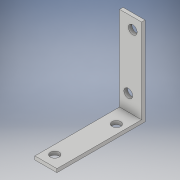
# Autodesk Inventor part: Plywood Pickle Mount Corner Bracket
Saved by Autodesk Inventor 2018 (Build 220112000, 112)
## iProperties
Created: 2018-02-14
Part Number: Plywood Pickle Mount Corner Bracket
Material: Generic
Document SubType Name: Modeling
Designer: owner
Density: 1 g/cm^3
Appearance: Default
Author: owner
Autodesk Inventor part; units mm, degrees
ref_plane "YZ Plane" through (0, 0, 0) normal (1, 0, 0) x (0, 1, 0)
ref_plane "XZ Plane" through (0, 0, 0) normal (0, 1, 0) x (-1, 0, 0)
ref_plane "XY Plane" through (0, 0, 0) normal (0, 0, 1) x (1, 0, 0)
sketch "Sketch1" plane through (0, 0, 0) normal (1, 0, 0) x (0, 1, 0)
  line L0 (0, 0) -> (0, -63.5)
  line L1 (0, -63.5) -> (63.5, -63.5)
  line L2 (63.5, -63.5) -> (63.5, -60.96)
  line L3 (0, 0) -> (2.54, 0)
  line L4 (2.54, 0) -> (2.54, -60.96)
  line L5 (2.54, -60.96) -> (63.5, -60.96)
  dimension "d0" = 63.5
  dimension "d1" = 63.5
  dimension "d2" = 2.54
  dimension "d3" = 2.54
  constraints: 12 end point, 3 perpendicular, 1 horizontal, 1 parallel, 1 vertical
  measures "d0" distance of L0.start L0.end
  measures "d1" distance of L0.end L1.end
  measures "d2" distance of L1.end L2.end
  measures "d3" distance of L0.start L3.end
extrude "Extrusion1" add sketch "Sketch1" along normal blind 15.875
sketch "Sketch2" plane through (0, 2.54, 0) normal (0, 1, 0) x (1, 0, 0)
  circle A0 centre (6.35, 7.9375) radius 3.175
  circle A1 centre (9.525, 49.2125) radius 3.175
  point P0 (0, 0)
  dimension "d6" = 6.35
  dimension "d7" = 6.35
  constraints: 2 centre point
  measures "d6" diameter of A0
  measures "d7" diameter of A1
extrude "Extrusion2" cut sketch "Sketch2" against normal through all contours A1
extrude "Extrusion3" cut sketch "Sketch2" against normal through all contours A0
sketch "Sketch3" plane through (0, 2.54, -60.96) normal (0, 0, 1) x (1, 0, 0)
  line L0 (15.875, 60.96) -> (15.875, 53.0225)
  line L1 (15.875, 53.0225) -> (9.525, 53.0225)
  line L2 (15.875, 53.0225) -> (15.875, 11.7475)
  line L3 (15.875, 11.7475) -> (6.35, 11.7475)
  circle A0 centre (6.35, 11.7475) radius 3.175
  circle A1 centre (9.525, 53.0225) radius 3.175
  point P0 (0, -2.54)
  dimension "d12" = 6.35
  dimension "d13" = 6.35
  dimension "d14" = 6.35
  dimension "d15" = 7.9375
  dimension "d16" = 41.275
  dimension "d17" = 9.525
  constraints: 8 end point, 2 centre point, 2 coincident, 2 horizontal
  measures "d12" diameter of A0
  measures "d13" diameter of A1
  measures "d14" distance of L0.end L1.end
  measures "d15" distance of L0.start L0.end
  measures "d16" distance of L0.end L2.end
  measures "d17" distance of L2.end L3.end
extrude "Extrusion4" cut sketch "Sketch3" against normal through all contours A0
extrude "Extrusion5" cut sketch "Sketch3" against normal through all contours A1
body "Solid1"
